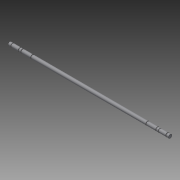
# Autodesk Inventor part: IDLER SHAFT
Saved by Autodesk Inventor 2014 (Build 180170000, 170)
## iProperties
Created: 2013-09-20
Part Number: IDLER SHAFT
Material: Generic
Document SubType Name: Modeling
Designer: Brandon
Density: 1 g/cm^3
Appearance: Default
Author: Brandon
Autodesk Inventor part; units mm, degrees
ref_plane "YZ Plane" through (0, 0, 0) normal (1, 0, 0) x (0, 1, 0)
ref_plane "XZ Plane" through (0, 0, 0) normal (0, 1, 0) x (-1, 0, 0)
ref_plane "XY Plane" through (0, 0, 0) normal (0, 0, 1) x (1, 0, 0)
sketch "Sketch1" plane through (0, 0, 0) normal (0, 1, 0) x (-1, 0, 0)
  line L0 (0, 0) -> (0, 5)
  line L1 (0, 0) -> (-24.5, 0) construction
  line L2 (-24.5, 0) -> (-28.5, 0) construction
  line L3 (-24.5, 0) -> (-20.5, 0) construction
  line L4 (-28.5, 0) -> (-29.75, 0) construction
  line L5 (-29.75, 0) -> (-32.75, 0) construction
  line L6 (-32.75, 0) -> (-34, 0) construction
  line L7 (-32.75, 0) -> (-32.85, 0) construction
  line L8 (-32.85, 0.65) -> (-32.95, 0.75)
  line L9 (-32.85, 0.65) -> (-32.75, 0.75)
  line L10 (-32.95, 0.75) -> (-34, 0.75)
  line L11 (-29.65, 0.65) -> (-29.55, 0.75)
  line L12 (-29.65, 0.65) -> (-29.75, 0.75)
  line L13 (-28.6, 0.65) -> (-28.5, 0.75)
  line L14 (-24.4, 0.65) -> (-24.3, 0.75)
  line L15 (-24.4, 0.65) -> (-24.5, 0.75)
  line L16 (-34, 0.75) -> (-34, 0)
  line L17 (0, 0.75) -> (-24.3, 0.75)
  line L18 (-24.5, 0.75) -> (-28.5, 0.75)
  line L19 (-29.75, 0.75) -> (-32.75, 0.75)
  line L20 (-34, 0) -> (0, 0)
  line L21 (-32.85, 0) -> (-32.85, 0.75) construction
  line L22 (-34, 0.65) -> (0, 0.65) construction
  line L23 (-29.65, 0) -> (-29.65, 0.75) construction
  line L24 (-28.6, 0) -> (-28.6, 0.7608) construction
  line L25 (-28.6, 0.65) -> (-28.7, 0.75)
  line L26 (-28.7, 0.75) -> (-29.55, 0.75)
  line L27 (-24.4, 0) -> (-24.4, 0.75) construction
  line L28 (0, 0) -> (24.5, 0) construction
  line L29 (24.5, 0) -> (28.5, 0) construction
  line L30 (24.5, 0) -> (20.5, 0) construction
  line L31 (28.5, 0) -> (29.75, 0) construction
  line L32 (29.75, 0) -> (32.75, 0) construction
  line L33 (32.75, 0) -> (34, 0) construction
  line L34 (32.75, 0) -> (32.85, 0) construction
  line L35 (32.85, 0.65) -> (32.95, 0.75)
  line L36 (32.85, 0.65) -> (32.75, 0.75)
  line L37 (32.95, 0.75) -> (34, 0.75)
  line L38 (29.65, 0.65) -> (29.55, 0.75)
  line L39 (29.65, 0.65) -> (29.75, 0.75)
  line L40 (28.6, 0.65) -> (28.5, 0.75)
  line L41 (24.4, 0.65) -> (24.5, 0.75)
  line L42 (24.4, 0.65) -> (24.3, 0.75)
  line L43 (34, 0.75) -> (34, 0)
  line L44 (0, 0.75) -> (24.3, 0.75)
  line L45 (24.5, 0.75) -> (28.5, 0.75)
  line L46 (29.75, 0.75) -> (32.75, 0.75)
  line L47 (34, 0) -> (0, 0)
  line L48 (32.85, 0) -> (32.85, 0.75) construction
  line L49 (34, 0.65) -> (0, 0.65) construction
  line L50 (29.65, 0) -> (29.65, 0.75) construction
  line L51 (28.6, 0) -> (28.6, 0.7608) construction
  line L52 (28.6, 0.65) -> (28.7, 0.75)
  line L53 (28.7, 0.75) -> (29.55, 0.75)
  line L54 (24.4, 0) -> (24.4, 0.75) construction
  dimension "d5" = 24.5
  dimension "d7" = 4
  dimension "d9" = 1.25
  dimension "d11" = 3
  dimension "d13" = 1.25
  dimension "d17" = 0.1
  dimension "d20" = 45
  dimension "d21" = 45
  dimension "d22" = 90
  dimension "d23" = 0.1
  dimension "d24" = 45
  dimension "d25" = 45
  dimension "d26" = 0.1
  dimension "d27" = 0.75
  dimension "d28" = 45
  dimension "d29" = 45
  dimension "d30" = 0.65
  dimension "d31" = 0.1
  dimension "d32" = 45
  dimension "d33" = 45
  constraints: 110 end point, 29 point on line, 28 symmetric about line, 8 collinear, 6 horizontal, 4 perpendicular, 3 vertical, 1 parallel
  measures "d5" distance of L0.start L1.end
  measures "d7" distance of L1.end L2.end
  measures "d9" distance of L2.end L4.end
  measures "d11" distance of L4.end L5.end
  measures "d13" distance of L5.end L6.end
  measures "d17" distance of L5.end L7.end
  measures "d20" angle of L21 L9
  measures "d21" angle of L21 L8
  measures "d22" angle of L20 L21
  measures "d23" distance from line of L4.end L23
  measures "d24" angle of L23 L11
  measures "d25" angle of L12 L23
  measures "d26" distance of L2.end L24.start
  measures "d27" distance of L10.end L6.end
  measures "d28" angle of L24 L25
  measures "d29" angle of L24 L13
  measures "d30" distance between parallel lines of L4 L22
  measures "d31" distance of L1.end L27.start
  measures "d32" angle of L27 L14
  measures "d33" angle of L27 L15
revolve "Revolution1" add sketch "Sketch1" angle 360 about axis through (0, 0, 0) along (1, 0, 0)
body "Solid1"
